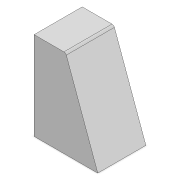
# Autodesk Inventor part: Part1
Saved by Autodesk Inventor 2020 (Build 240168000, 168)
## iProperties
Created: 2019-07-02
Part Number: Part1
Material: Generic
Document SubType Name: Modeling
Designer: chitl
Density: 1 g/cm^3
Appearance: Default
Author: chitl
Autodesk Inventor part; units mm, degrees
ref_plane "YZ Plane" through (0, 0, 0) normal (1, 0, 0) x (0, 1, 0)
ref_plane "XZ Plane" through (0, 0, 0) normal (0, 1, 0) x (-1, 0, 0)
ref_plane "XY Plane" through (0, 0, 0) normal (0, 0, 1) x (1, 0, 0)
sketch "Sketch1" plane through (0, 0, 0) normal (0, 0, 1) x (1, 0, 0)
  line L0 (-19.7993, 68.1553) -> (17.5761, 68.1553)
  line L1 (20.5597, 66.0662) -> (62.3445, -48.7367)
  line L2 (-19.7993, 68.1553) -> (-19.7993, -48.7367)
  line L3 (-19.7993, -48.7367) -> (62.3445, -48.7367)
  arc A0 (20.5597, 66.0662) -> (17.5761, 68.1553) centre (17.5761, 64.9803) ccw
  point P0 (0, 0)
  point P1 (19.7993, 68.1553)
  dimension "d0" = 110
  dimension "d1" = 39.5986
  dimension "d2" = 3.175
  dimension "d3" = 122.1707
  constraints: 8 end point, 2 point on circle, 2 point on line, 2 tangent, 1 centre point, 1 horizontal, 1 perpendicular, 1 vertical
  measures "d0" angle of L0 L1
  measures "d1" distance of L0.start point (19.799, 68.155)
  measures "d2" radius of A0
  measures "d3" distance of L1.start L1.end
extrude "Extrusion1" add sketch "Sketch1" along normal blind 63.5
sketch "Sketch2" plane through (-19.7993, -48.7367, 0) normal (-1, 0, 0) x (0, 0, 1)
  line L0 (10.7282, 97.9332) -> (52.7214, 97.9332)
  line L1 (52.7214, 97.9332) -> (52.7214, 3.0652)
  line L2 (52.7214, 3.0652) -> (10.7282, 3.0652)
  line L3 (10.7282, 3.0652) -> (10.7282, 97.9332)
  point P0 (0, 48.7367)
  constraints: 8 end point, 2 parallel, 1 horizontal, 1 perpendicular
extrude "Extrusion2" cut sketch "Sketch2" against normal blind 34.925
move faces "Move1" translate (0, 0, -6.35) faces at (21.035, -10.4691, 63.5)
move faces "Move2" translate (0, 0, 4.7752) faces at (21.035, -10.4691, 0)
move faces "Move3" translate (0, 6.35, 0) faces at (7.582, -48.7367, 22.2335)
move faces "Move4" translate (0, 0, 7.9502) faces at (20.2646, -6.2358, 57.15)
body "Solid1"
